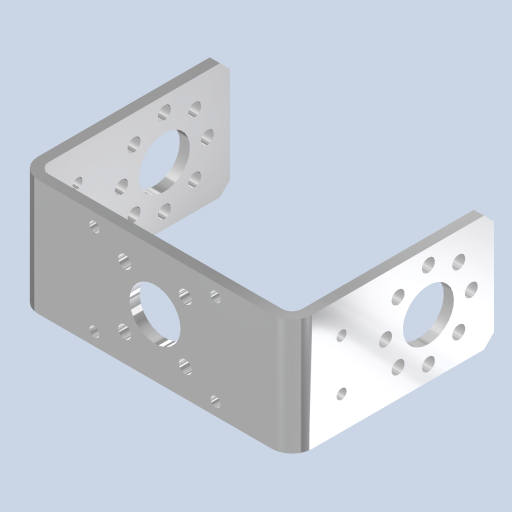
# Autodesk Inventor part: servo_arm_1170
Saved by Autodesk Inventor 2023 (Build 270158000, 158)
## iProperties
Created: 2015-11-25
Part Number: servo_arm_1170
Material: アルミニウム 5052
Document SubType Name: シート メタル
Designer: hiroaki
Density: 2.68 g/cm^3
Appearance: アルミニウム - フラット
Sheet Metal Rule: Default_mm
Flat Pattern Width: 2.3 cm
Flat Pattern Length: 12.7348 cm
Flat Pattern Area: 29.29 cm^2
Sheet Metal Width: 23.000 mm
Sheet Metal Length: 127.348 mm
Sheet Metal Area: 2928.999 mm^2
Mass: 11.4104 g
Surface Area: 52.5179 cm^2
Volume: 4.25761 cm^3
Author: hiroaki
Autodesk Inventor part; units mm, degrees
ref_plane "YZ Plane" through (0, 0, 0) normal (1, 0, 0) x (0, 1, 0)
ref_plane "XZ Plane" through (0, 0, 0) normal (0, 1, 0) x (-1, 0, 0)
ref_plane "XY Plane" through (0, 0, 0) normal (0, 0, 1) x (1, 0, 0)
sketch "スケッチ1" plane through (0, 0, 0) normal (0, 0, 1) x (1, 0, 0)
  line L0 (-27.15, 15) -> (-27.15, -15)
  line L1 (-27.15, -15) -> (27.15, -15)
  line L2 (27.15, -15) -> (27.15, 15)
  line L3 (27.15, 15) -> (25.15, 15)
  line L4 (25.15, 15) -> (25.15, -13)
  line L5 (25.15, -13) -> (-25.15, -13)
  line L6 (-25.15, -13) -> (-25.15, 15)
  line L7 (-25.15, 15) -> (-27.15, 15)
  point P0 (0, 0)
  point P1 (0, -13)
  point P2 (27.15, 0)
  dimension "d0" = 2
  dimension "d1" = 2
  dimension "d2" = 50.3
  dimension "d3" = 30
  constraints: 16 end point, 6 perpendicular, 2 equal length, 2 midpoint, 2 vertical, 1 horizontal alignment, 1 vertical alignment
  measures "d0" distance of L6.end L0.start
  measures "d1" distance between parallel lines of L5 L1
  measures "d2" distance of L4.end L5.end
  measures "d3" distance of L0.start L0.end
extrude "押し出し1" add sketch "スケッチ1" along normal blind 23
sketch "スケッチ3" plane through (-27.15, -15, 0) normal (0, -1, 0) x (1, 0, 0)
  line L0 (0, 23) -> (54.3, 23) projected
  line L1 (0, 0) -> (0, 23) projected
  circle A0 centre (27.15, 11.5) radius 5.05
  circle A1 centre (21.1396, 17.5104) radius 1.3
  circle A2 centre (27.15, 11.5) radius 8.5 construction
  line L2 (27.15, 11.5) -> (21.1396, 17.5104) construction
  line L3 (27.15, 11.5) -> (27.15, 18.5) construction
  circle A3 centre (15.15, 2.5) radius 1
  line L4 (27.15, 11.5) -> (20.15, 11.5) construction
  circle A4 centre (15.15, 20.5) radius 1
  circle A5 centre (39.15, 2.5) radius 1
  circle A6 centre (39.15, 20.5) radius 1
  circle A7 centre (21.1396, 5.4896) radius 1.3
  circle A8 centre (33.1604, 5.4896) radius 1.3
  circle A9 centre (33.1604, 17.5104) radius 1.3
  point P0 (27.15, 0)
  point P1 (0, 11.5)
  point P2 (27.15, 23)
  dimension "d25" = 17
  dimension "d22" = 10.1
  dimension "d24" = 7
  dimension "d26" = 2.6
  dimension "d27" = 45
  dimension "d32" = 2
  dimension "d33" = 9
  dimension "d34" = 12
  dimension "d55" = 360
  constraints: 9 centre point, 6 end point, 3 symmetric about line, 2 midpoint, 2 vertical alignment, 1 coincident, 1 horizontal, 1 horizontal alignment, 1 vertical, 15 other
  measures "d22" diameter of A0
  measures "d24" distance of L3.end A0.centre
  measures "d26" diameter of A1
  measures "d27" angle of L3 L2
  measures "d32" diameter of A3
  measures "d33" vertical distance of A0.centre A3.centre
  measures "d34" horizontal distance of A0.centre A3.centre
extrude "押し出し3" cut sketch "スケッチ3" against normal through all
sketch "スケッチ4" plane through (0, 0, 23) normal (0, 0, 1) x (1, 0, 0)
  line L0 (-27.15, 15) -> (-27.15, -15) projected
  line L1 (27.15, -15) -> (27.15, 15) projected
  line L2 (25.15, -13) -> (-25.15, -13) projected
  line L3 (-27.15, 33.5217) -> (27.15, 33.5217)
  line L4 (27.15, 33.5217) -> (27.15, -13)
  line L5 (27.15, -13) -> (-27.15, -13)
  line L6 (-27.15, -13) -> (-27.15, 33.5217)
  point P0 (-27.15, 13)
  point P1 (27.15, 13)
  point P2 (0, 0)
  constraints: 8 end point, 3 collinear, 2 parallel, 1 horizontal, 1 perpendicular
extrude "押し出し4" cut sketch "スケッチ4" against normal blind 100
sketch "スケッチ5" plane through (-25.15, -15, 23) normal (-1, 0, 0) x (0, -1, 0)
  line L0 (0, -23) -> (0, 0)
  line L1 (0, 0) -> (-40, 0)
  line L2 (-40, 0) -> (-40, -23)
  line L3 (-40, -23) -> (0, -23)
  constraints: 4 end point, 4 other
edge flange "フランジ1" height 40 angle 90 thickness 2 bend radius 2 thickness toward (-1, 0, 0) relief tear relief width 2 relief depth 1 corner gap 2 corner form 0 edges at (-27.15, -13, 11.5) (27.15, -13, 11.5) wall of the first edge with corners at (-25.15, -15, 0) (-25.15, -15, 23) (-25.15, 25, 23) (-25.15, 25, 0)
bend "曲げ1"
corner "コーナー1"
sketch "スケッチ2" plane through (27.15, -15, 0) normal (1, 0, 0) x (0, 0, -1)
  line L0 (0, 30) -> (-23, 30) projected
  line L1 (0, 0) -> (-23, 0) projected
  circle A0 centre (-11.5, 27) radius 5.05
  circle A1 centre (-20, 27) radius 1.3
  circle A2 centre (-17.5104, 20.9896) radius 1.3
  circle A3 centre (-11.5, 18.5) radius 1.3
  circle A4 centre (-5.4896, 20.9896) radius 1.3
  circle A5 centre (-3, 27) radius 1.3
  circle A6 centre (-5.4896, 33.0104) radius 1.3
  circle A7 centre (-11.5, 35.5) radius 1.3
  circle A8 centre (-17.5104, 33.0104) radius 1.3
  circle A9 centre (-16.5, 9.8) radius 1
  line L2 (-11.5, 27) -> (-11.5, 30) construction
  circle A10 centre (-6.5, 9.8) radius 1
  point P0 (0, 15)
  point P1 (-16.55, 27)
  point P2 (-6.45, 27)
  dimension "d6" = 27
  dimension "d7" = 8.5
  dimension "d8" = 2.6
  dimension "d9" = 5.05
  dimension "d12" = 360
  dimension "d14" = 2
  dimension "d16" = 9.8
  constraints: 11 centre point, 2 end point, 2 horizontal alignment, 2 point on circle, 1 midpoint, 1 symmetric about line, 1 vertical, 1 vertical alignment, 18 other
  measures "d6" distance from line of L1 A1.centre
  measures "d7" distance of L2.start A1.centre
  measures "d8" diameter of A1
  measures "d9" radius of A0
  measures "d14" diameter of A9
  measures "d16" distance from line of L1 A9.centre
extrude "押し出し2" cut sketch "スケッチ2" against normal blind 100
chamfer "面取り2" distance 2 angle 45 4 edges at (-26.15, 25, 23) (-26.15, 25, 0) (26.15, 25, 23) (26.15, 25, 0)
equation "\"d1\" = d0"
equation "\"d39\" = BendReliefWidth"
equation "\"d40\" = BendReliefDepth"
equation "\"d41\" = MinimumRemnant"
equation "\"d42\" = BendRadius"
equation "\"d45\" = BendRadius"
equation "\"d46\" = CornerReliefSize"
equation "\"d47\" = GapSize"
equation "\"d48\" = JacobiRadiusSize"
equation "\"d52\" = Thickness"
equation "\"BendRadius\" = Thickness"
equation "\"BendReliefWidth\" = Thickness"
equation "\"BendReliefDepth\" = 0.5 * Thickness"
equation "\"CornerReliefSize\" = 4 * Thickness"
equation "\"MinimumRemnant\" = 2 * Thickness"
equation "\"TransitionRadius\" = BendRadius"
equation "\"JacobiRadiusSize\" = BendRadius"
equation "\"GapSize\" = Thickness"
equation "\"Thickness\" = 2"
